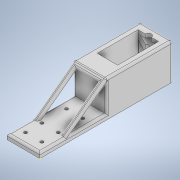
# Autodesk Inventor part: soporte_servo
Saved by Autodesk Inventor 2021 (Build 250183000, 183)
## iProperties
Created: 2021-10-04
Part Number: soporte_servo
Material: Genérico
Document SubType Name: Modeling
Designer: Joaquín
Density: 1 g/cm^3
Appearance: Valor por defecto
Author: Joaquín
Autodesk Inventor part; units mm, degrees
ref_plane "YZ Plane" through (0, 0, 0) normal (1, 0, 0) x (0, 1, 0)
ref_plane "XZ Plane" through (0, 0, 0) normal (0, 1, 0) x (-1, 0, 0)
ref_plane "XY Plane" through (0, 0, 0) normal (0, 0, 1) x (1, 0, 0)
sketch "Boceto1" plane through (0, 0, 0) normal (0, 1, 0) x (-1, 0, 0)
  line L0 (0, 0) -> (32, 0)
  line L1 (32, 0) -> (32, -80)
  line L2 (32, -80) -> (0, -80)
  line L3 (0, -80) -> (0, 0)
  line L4 (32, 0) -> (32, -10)
  line L5 (32, -10) -> (32, -20)
  line L6 (0, 0) -> (0, -10)
  line L7 (0, -10) -> (0, -20)
  line L8 (32, -80) -> (32, -70)
  line L9 (0, -80) -> (0, -70)
  line L10 (32, 0) -> (0, 0)
  constraints: 22 end point, 6 point on line, 2 perpendicular, 1 collinear, 1 horizontal
extrude "Extrusión1" add sketch "Boceto1" along normal blind 5
sketch "Boceto3" plane through (0, 0, 0) normal (1, 0, 0) x (0, 0, -1)
  line L0 (0, 5) -> (80, 5) projected
  line L1 (80, 5) -> (80, 0)
  line L2 (80, 0) -> (130, 0)
  line L3 (130, 0) -> (130, 45)
  line L4 (130, 45) -> (80, 45)
  line L5 (80, 45) -> (80, 5)
  line L6 (80, 0) -> (80, 5) projected
  line L7 (0, 5) -> (80, 5)
  line L8 (80, 45) -> (65, 45)
  line L9 (0, 5) -> (25, 5)
  line L10 (25, 5) -> (65, 45)
  point P0 (0, 0)
  dimension "d33" = 50
  dimension "d35" = 50
  dimension "d37" = 15
  dimension "d38" = 25
  constraints: 18 end point, 2 horizontal, 2 perpendicular, 2 vertical, 1 point on line
  measures "d33" distance of L1.end L2.end
  measures "d35" distance of L3.end L4.end
  measures "d37" distance of L4.end L8.end
  measures "d38" distance of L0.start L9.end
extrude "Extrusión3" add sketch "Boceto3" against normal blind 32
sketch "Boceto4" plane through (-10, 5, -70) normal (0, -1, 0) x (1, 0, 0)
  circle A0 centre (0, 0) radius 1.5
  circle A1 centre (-12, 0) radius 1.5 projected
  circle A2 centre (-12, 0) radius 1.5
  point P0 (10, 70)
  constraints: 2 centre point, 1 coincident
extrude "Extrusión4" [suppressed]
sketch "Boceto8" plane through (0, 0, 0) normal (0, -1, 0) x (1, 0, 0)
  line L0 (-6, -125) -> (-26, -125)
  line L1 (-6, -85) -> (-6, -125)
  line L2 (-26, -85) -> (-26, -125)
  line L3 (-6, -85) -> (-26, -85)
  constraints: 8 end point, 2 perpendicular, 1 horizontal
extrude "Extrusión8" cut sketch "Boceto8" against normal blind 40
sketch "Boceto9" plane through (-32, 0, 0) normal (-1, 0, 0) x (0, 0, 1)
  line L0 (-65, 45) -> (-130, 45) projected
  line L1 (-130, 45) -> (-130, 35)
  line L2 (-130, 45) -> (-130, 0) projected
  line L3 (-35, 5) -> (-65, 35) projected
  line L4 (-130, 35) -> (-65, 35)
  line L5 (-65, 35) -> (-65, 45) projected
  line L6 (-65, 35) -> (-65, 45)
  line L7 (-65, 45) -> (-25, 5) projected
  line L8 (-65, 45) -> (-130.7928, 45)
  point P0 (0, 0)
  dimension "d76" = 10
  constraints: 8 end point, 2 point on line, 1 collinear
  measures "d76" distance of L0.end L1.end
extrude "Extrusión9" cut sketch "Boceto9" against normal blind 40
sketch "Boceto10" plane through (-32, 0, 0) normal (-1, 0, 0) x (0, 0, 1)
  line L0 (-65, 35) -> (-65, 45) projected
  line L1 (-65, 35) -> (-55, 35)
  line L2 (-65, 45) -> (-25, 5) projected
  line L3 (-65, 45) -> (-65, 35)
  line L4 (-65, 45) -> (-55, 35)
  point P0 (0, 0)
  constraints: 6 end point, 1 collinear, 1 horizontal, 1 perpendicular, 1 point on line
extrude "Extrusión10" cut sketch "Boceto10" against normal blind 40
sketch "Boceto11" plane through (-32, 0, 0) normal (-1, 0, 0) x (0, 0, 1)
  line L0 (-55, 35) -> (-130, 35) projected
  line L1 (-55, 35) -> (-65, 35)
  line L2 (-65, 35) -> (-25, 5)
  line L3 (-25, 5) -> (-55, 35) projected
  line L4 (-25, 5) -> (-55, 35)
  point P0 (0, 0)
  dimension "d81" = 10
  constraints: 6 end point, 1 collinear, 1 point on line
  measures "d81" distance of L0.start L1.end
extrude "Extrusión11" cut sketch "Boceto11" against normal blind 40
sketch "Boceto13" plane through (0, 0, 0) normal (1, 0, 0) x (0, 0, -1)
  line L0 (65, 25) -> (65, 5)
  line L1 (65, 5) -> (35, 5)
  line L2 (65, 25) -> (65, 30)
  line L3 (35, 5) -> (30, 5)
  line L4 (30, 5) -> (65, 30)
  line L5 (130, 0) -> (130, 35) projected
  line L6 (85, 0) -> (125, 0) projected
  line L7 (90, 30) -> (120, 30)
  line L8 (125, 25) -> (125, 10)
  line L9 (120, 5) -> (90, 5)
  line L10 (85, 10) -> (85, 25)
  line L11 (98.125, 17.5) -> (85, 25)
  line L12 (98.125, 17.5) -> (85, 10)
  line L13 (105, 13.5714) -> (90, 5)
  line L14 (105, 13.5714) -> (120, 5)
  line L15 (111.875, 17.5) -> (125, 10)
  line L16 (111.875, 17.5) -> (125, 25)
  line L17 (105, 21.4286) -> (120, 30)
  line L18 (105, 21.4286) -> (90, 30)
  point P0 (0, 0)
  point P1 (25, 5)
  dimension "d89" = 5
  dimension "d90" = 5
  constraints: 34 end point, 3 horizontal, 1 perpendicular, 1 vertical
  measures "d89" distance of L0.start L2.end
  measures "d90" distance of L1.end L3.end
extrude "Extrusión13" cut sketch "Boceto13" against normal blind 40 contours L0 L1 L3 L4 L2
sketch "Boceto20" plane through (0, 5, -65) normal (0, 0, 1) x (1, 0, 0)
  line L0 (-27, 7.5) -> (-27, 0)
  line L1 (0, 0) -> (-32, 0) projected
  line L2 (-5, 17.5) -> (-5, 7.5) projected
  line L3 (-5, 17.5) -> (-5, 25)
  line L4 (0, 25) -> (-32, 25) projected
  line L5 (-5, 25) -> (-27, 25)
  line L6 (-27, 25) -> (-27, 0)
  line L7 (-27, 0) -> (-5, 0)
  line L8 (-5, 0) -> (-5, 25)
  point P0 (0, -5)
  point P1 (-5, 0)
  constraints: 12 end point, 2 parallel, 2 point on line, 2 vertical, 1 horizontal, 1 perpendicular
extrude "Extrusión15" cut sketch "Boceto20" along normal blind 400
fillet "Empalme1" radius 2 19 edges at (-32, 5, -47.5) (-32, 5, -12.5) (-32, 20, -45) (-27, 17.5, -41.6667) (-27, 17.5, -47.5) (-32, 17.5, -47.5) (-5, 17.5, -41.6667) (-5, 17.5, -47.5) (0, 20, -45) (0, 17.5, -47.5) (0, 5, -12.5) (0, 5, -47.5) (-16, 5, 0) (-32, 17.5, -65) (0, 17.5, -65) (-16, 30, -58.3333) (-16, 35, -65) (0, 35, -97.5) (-32, 35, -97.5)
sketch "Boceto24" plane through (-30, 35, -65.6667) normal (0, 1, 0) x (1, 0, 0)
  circle A0 centre (14, 19.3333) radius 3
  point P0 (30, -65.6667)
  point P1 (24, 19.3333)
  constraints: 1 centre point
extrude "Extrusión18" cut sketch "Boceto24" against normal blind 39
fillet "Empalme2" radius 2 5 edges at (-16, 35, -130) (-0.5858, 34.4142, -130) (0, 16.5, -130) (-31.4142, 34.4142, -130) (-32, 16.5, -130)
sketch "Boceto25" plane through (0, 0, 0) normal (0, -1, 0) x (1, 0, 0)
  line L0 (-26, -125) -> (-26, -85) projected
  line L1 (-6, -85) -> (-6, -125) projected
  line L2 (-26, -125) -> (-6, -125)
  line L3 (-6, -125) -> (-6, -85)
  arc A0 (-13, -85) -> (-19, -85) centre (-16, -85) ccw projected
  line L4 (-6, -85) -> (-13, -85)
  point P0 (0, 0)
  constraints: 6 end point, 1 collinear, 1 horizontal, 1 perpendicular
sketch "Boceto22" plane through (0, 0, -130) normal (0, 0, -1) x (-1, 0, 0)
  line L0 (8.3738, 31.3099) -> (23.6262, 31.3099)
  line L1 (25.6262, 26.3099) -> (25.6262, 8.6901)
  line L2 (23.5, 3.6901) -> (8.3738, 3.6901)
  line L3 (6.3738, 8.6901) -> (6.3738, 26.3099)
  line L4 (8.3738, 31.3099) -> (16, 22.7922)
  line L5 (17.7383, 17.5) -> (25.6262, 8.6901)
  line L6 (6.3738, 8.6901) -> (14.237, 17.4725)
  line L7 (16, 22.7922) -> (23.6262, 31.3099)
  line L8 (23.5, 3.6901) -> (15.9606, 12.1637)
  line L9 (14.237, 17.4725) -> (6.3738, 26.3099)
  line L10 (8.3738, 3.6901) -> (15.9606, 12.1637)
  line L11 (17.7383, 17.5) -> (25.6262, 26.3099)
  point P0 (0, 0)
  point P1 (0, 35)
  point P2 (32, 35)
  constraints: 24 end point, 2 parallel, 1 horizontal, 1 perpendicular
extrude "Extrusión16" cut sketch "Boceto22" against normal blind 1
sketch "Boceto26" plane through (0, 0, 0) normal (0, -1, 0) x (1, 0, 0)
  line L0 (-13, -85) -> (-6, -85) projected
  line L1 (-6, -85) -> (-6, -82)
  line L2 (-6, -82) -> (-16, -82)
  arc A0 (-13, -85) -> (-19, -85) centre (-16, -85) ccw projected
  line L3 (-26, -85) -> (-26, -82)
  line L4 (-26, -82) -> (-16, -82)
  arc A1 (-13, -85) -> (-19, -85) centre (-16, -85) ccw
  line L5 (-26, -85) -> (-19, -85)
  line L6 (-13, -85) -> (-6, -85)
  line L7 (-26, -125) -> (-16, -125)
  line L8 (-23.5, -125) -> (-15.9606, -125) projected
  line L9 (-16, -125) -> (-16, -122)
  arc A2 (-19, -122) -> (-13, -122) centre (-16, -122) ccw
  line L10 (-26, -125) -> (-26, -85) projected
  line L11 (-26, -122) -> (-19, -122)
  line L12 (-13, -122) -> (-6, -122)
  point P0 (0, 0)
  dimension "d187" = 3
  dimension "d188" = 10
  dimension "d189" = 3
  dimension "d190" = 6
  constraints: 20 end point, 5 point on circle, 4 perpendicular, 3 point on line, 2 centre point, 2 coincident, 2 horizontal, 1 collinear, 1 tangent, 1 vertical
  measures "d187" distance of L0.end L1.end
  measures "d188" distance of L7.start L7.end
  measures "d189" distance of L7.end L9.end
  measures "d190" diameter of A2
sketch "Boceto27" plane through (0, 0, 0) normal (0, -1, 0) x (1, 0, 0)
  line L0 (-26, -125) -> (-26, -85) projected
  line L1 (-26, -125) -> (-26, -122)
  line L2 (-26, -122) -> (-19, -122)
  line L3 (-19, -122) -> (-13, -122)
  line L4 (-13, -122) -> (-6, -122)
  line L5 (-6, -85) -> (-6, -125) projected
  line L6 (-6, -125) -> (-6, -122)
  line L7 (-6, -125) -> (-26, -125)
  arc A0 (-19, -122) -> (-13, -122) centre (-16, -122) ccw
  point P0 (0, 0)
  point P1 (-16, -125)
  dimension "d191" = 3
  dimension "d192" = 7
  dimension "d193" = 6
  constraints: 12 end point, 4 point on line, 2 perpendicular, 2 point on circle, 1 centre point, 1 collinear, 1 midpoint
  measures "d191" distance of L0.start L1.end
  measures "d192" distance of L1.end L2.end
  measures "d193" distance of L2.end L3.end
extrude "Extrusión19" cut sketch "Boceto26" against normal blind 100 contours A0 L2 L1 L0 | A0 L5 L3 L4
extrude "Extrusión20" add sketch "Boceto27" against normal blind 35 contours L0 L2 A0 L7 | A0 L4 L5 L7
sketch "Boceto28" plane through (-2, 0, -130) normal (0, 0, -1) x (-1, 0, 0)
  line L0 (14, 22.7922) -> (6.3738, 31.3099) projected
  line L1 (6.3738, 31.3099) -> (21.6262, 31.3099)
  line L2 (21.6262, 31.3099) -> (14, 22.7922) projected
  line L3 (21.6262, 31.3099) -> (14, 22.7922)
  line L4 (14, 22.7922) -> (6.3738, 31.3099)
  line L5 (4.3738, 26.3099) -> (12.237, 17.4725) projected
  line L6 (12.237, 17.4725) -> (4.3738, 26.3099)
  line L7 (4.3738, 8.6901) -> (12.237, 17.4725) projected
  line L8 (4.3738, 26.3099) -> (4.3738, 8.6901)
  line L9 (4.3738, 8.6901) -> (12.237, 17.4725)
  line L10 (15.7383, 17.5) -> (23.6262, 26.3099) projected
  line L11 (15.7383, 17.5) -> (23.6262, 26.3099)
  line L12 (23.6262, 26.3099) -> (23.6262, 8.6901) projected
  line L13 (23.6262, 26.3099) -> (23.6262, 8.6901)
  line L14 (23.6262, 8.6901) -> (15.7383, 17.5)
  line L15 (6.3738, 3.6901) -> (14, 3.6901) projected
  line L16 (14, 12.1194) -> (6.3738, 3.6901)
  line L17 (14, 12.1194) -> (21.5, 3.6901)
  line L18 (21.5, 5) -> (21.5, 0) projected
  line L19 (14, 3.6901) -> (21.5, 3.6901) projected
  line L20 (6.3738, 3.6901) -> (21.5, 3.6901)
  point P0 (-2, 0)
  constraints: 24 end point, 6 collinear, 1 point on line, 1 vertical
extrude "Extrusión21" cut sketch "Boceto28" against normal blind 35
sketch "Boceto29" plane through (0, 0, 0) normal (0, -1, 0) x (1, 0, 0)
  circle A0 centre (-8, -10) radius 1.5
  circle A1 centre (-24, -10) radius 1.5
  circle A2 centre (-24, -26) radius 1.5
  circle A3 centre (-8, -26) radius 1.5
  circle A4 centre (-8, -50) radius 1.5
  circle A5 centre (-24, -50) radius 1.5
  dimension "d224" = 3
  dimension "d225" = 3
  dimension "d226" = 3
  dimension "d227" = 3
  dimension "d228" = 3
  dimension "d229" = 3
  constraints: 6 centre point
  measures "d224" diameter of A0
  measures "d225" diameter of A1
  measures "d226" diameter of A2
  measures "d227" diameter of A3
  measures "d228" diameter of A4
  measures "d229" diameter of A5
extrude "Extrusión22" cut sketch "Boceto29" against normal blind 10
